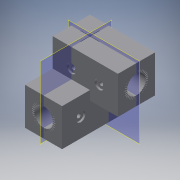
# Autodesk Inventor part: cam_holder_angle_part
Saved by Autodesk Inventor 2019 (Build 230136000, 136)
## iProperties
Created: 2024-08-06
Part Number: cam_holder_angle_part
Material: Generisch
Document SubType Name: Modeling
Designer: nic
Density: 1 g/cm^3
Appearance: Vorgabe
Author: nic
Autodesk Inventor part; units mm, degrees
ref_plane "YZ Plane" through (0, 0, 0) normal (1, 0, 0) x (0, 1, 0)
ref_plane "XZ Plane" through (0, 0, 0) normal (0, 1, 0) x (-1, 0, 0)
ref_plane "XY Plane" through (0, 0, 0) normal (0, 0, 1) x (1, 0, 0)
sketch "Skizze12" plane through (0, 0, 0) normal (0, 0, 1) x (1, 0, 0)
  circle A0 centre (0, 0) radius 10.1
  line L0 (-20, 20) -> (20, 20)
  line L1 (20, 20) -> (20, -20)
  line L2 (20, -20) -> (-20, -20)
  line L3 (-20, -20) -> (-20, 20)
  line L4 (-20, 20) -> (20, -20) construction
  line L5 (20, 20) -> (-20, -20) construction
  dimension "d59" = 20.2
  dimension "d60" = 40
  dimension "d61" = 40
  constraints: 12 end point, 2 midpoint, 2 parallel, 1 centre point, 1 coincident, 1 horizontal, 1 perpendicular
  measures "d59" diameter of A0
  measures "d60" distance of L1.end L2.end
  measures "d61" distance of L0.end L1.end
extrude "Extrusion10" add sketch "Skizze12" along normal blind 70
sketch "Skizze13" plane through (-20, -20, 0) normal (-1, 0, 0) x (0, 0, 1)
  line L0 (70, 30.1) -> (70, 9.9) projected
  line L1 (0, 9.9) -> (0, 30.1) projected
  line L2 (0, 30.1) -> (40, 30.1)
  line L3 (40, 30.1) -> (40, 70.1)
  line L4 (40, 70.1) -> (0, 70.1)
  line L5 (0, 70.1) -> (0, 30.1)
  circle A0 centre (20, 50.1) radius 10.1
  point P0 (0, 20)
  dimension "d64" = 40
  dimension "d65" = 40
  dimension "d66" = 20.2
  constraints: 8 end point, 2 parallel, 1 centre point, 1 horizontal, 1 perpendicular
  measures "d64" distance of L4.end L3.end
  measures "d65" distance of L3.end L2.end
  measures "d66" diameter of A0
extrude "Extrusion11" add sketch "Skizze13" against normal blind 70
sketch "Skizze14" plane through (-20, 20, 40) normal (0, 0, 1) x (1, 0, 0)
  line L0 (70, 20.2) -> (70, 0) projected
  line L1 (0, 0) -> (0, 20.2) projected
  line L2 (0, 0) -> (0, 20.2) projected
  line L3 (0, 10.1) -> (20, 10.1)
  line L4 (70, 20.2) -> (70, 0) projected
  line L5 (70, 10.1) -> (50, 10.1)
  point P0 (20, -20)
  dimension "d69" = 20
  dimension "d70" = 20
  constraints: 4 end point, 2 coincident, 2 midpoint, 1 horizontal, 1 point on line
  measures "d69" distance of L3.start L3.end
  measures "d70" distance of L5.start L5.end
hole "Bohrung3" at (0, 30.1, 40) at (30, 30.1, 40) direction (0, 0, -1) diameter 4.3 depth 12 tip angle 118 counterbore diameter 10 counterbore depth 2
sketch "Skizze15" plane through (20, -20, 70) normal (1, 0, 0) x (0, 0, -1)
  line L0 (0, 9.9) -> (0, 30.1) projected
  line L1 (70, 30.1) -> (70, 9.9) projected
  line L2 (0, 9.9) -> (0, 30.1) projected
  line L3 (0, 20) -> (20, 20)
  line L4 (70, 20) -> (50, 20)
  dimension "d78" = 20
  dimension "d79" = 20
  constraints: 4 end point, 2 coincident, 2 horizontal, 1 midpoint
  measures "d78" distance of L3.start L3.end
  measures "d79" distance of L4.start L4.end
hole "Bohrung4" at (20, 0, 50) at (20, 0, 20) direction (-1, 0, 0) diameter 4.3 depth 12 tip angle 118 counterbore diameter 10 counterbore depth 2
sketch "Skizze16" plane through (50, -20, 0) normal (1, 0, 0) x (0, 0, -1)
  circle A0 centre (-20, 50.1) radius 10.1 construction
  line L0 (-20.25, 57.7) -> (-19.75, 57.7)
  line L1 (-19.75, 57.7) -> (-19.75, 62.7)
  line L2 (-19.75, 62.7) -> (-20.25, 62.7)
  line L3 (-20.25, 62.7) -> (-20.25, 57.7)
  line L4 (-20.25, 57.7) -> (-19.75, 62.7) construction
  line L5 (-19.75, 57.7) -> (-20.25, 62.7) construction
  line L6 (-21.5659, 57.5411) -> (-21.0735, 57.628)
  line L7 (-21.0735, 57.628) -> (-21.9418, 62.552)
  line L8 (-21.9418, 62.552) -> (-22.4342, 62.4652)
  line L9 (-22.4342, 62.4652) -> (-21.5659, 57.5411)
  line L10 (-21.5659, 57.5411) -> (-21.9418, 62.552) construction
  line L11 (-21.0735, 57.628) -> (-22.4342, 62.4652) construction
  line L12 (-22.8343, 57.1562) -> (-22.3644, 57.3272)
  line L13 (-22.3644, 57.3272) -> (-24.0745, 62.0256)
  line L14 (-24.0745, 62.0256) -> (-24.5444, 61.8546)
  line L15 (-24.5444, 61.8546) -> (-22.8343, 57.1562)
  line L16 (-22.8343, 57.1562) -> (-24.0745, 62.0256) construction
  line L17 (-22.3644, 57.3272) -> (-24.5444, 61.8546) construction
  line L18 (-24.0165, 56.5568) -> (-23.5835, 56.8068)
  line L19 (-23.5835, 56.8068) -> (-26.0835, 61.1369)
  line L20 (-26.0835, 61.1369) -> (-26.5165, 60.8869)
  line L21 (-26.5165, 60.8869) -> (-24.0165, 56.5568)
  line L22 (-24.0165, 56.5568) -> (-26.0835, 61.1369) construction
  line L23 (-23.5835, 56.8068) -> (-26.5165, 60.8869) construction
  line L24 (-25.0767, 55.7612) -> (-24.6937, 56.0826)
  line L25 (-24.6937, 56.0826) -> (-27.9076, 59.9129)
  line L26 (-27.9076, 59.9129) -> (-28.2906, 59.5915)
  line L27 (-28.2906, 59.5915) -> (-25.0767, 55.7612)
  line L28 (-25.0767, 55.7612) -> (-27.9076, 59.9129) construction
  line L29 (-24.6937, 56.0826) -> (-28.2906, 59.5915) construction
  line L30 (-25.9826, 54.7937) -> (-25.6612, 55.1767)
  line L31 (-25.6612, 55.1767) -> (-29.4915, 58.3906)
  line L32 (-29.4915, 58.3906) -> (-29.8129, 58.0076)
  line L33 (-29.8129, 58.0076) -> (-25.9826, 54.7937)
  line L34 (-25.9826, 54.7937) -> (-29.4915, 58.3906) construction
  line L35 (-25.6612, 55.1767) -> (-29.8129, 58.0076) construction
  line L36 (-26.7068, 53.6835) -> (-26.4568, 54.1165)
  line L37 (-26.4568, 54.1165) -> (-30.7869, 56.6165)
  line L38 (-30.7869, 56.6165) -> (-31.0369, 56.1835)
  line L39 (-31.0369, 56.1835) -> (-26.7068, 53.6835)
  line L40 (-26.7068, 53.6835) -> (-30.7869, 56.6165) construction
  line L41 (-26.4568, 54.1165) -> (-31.0369, 56.1835) construction
  line L42 (-27.2272, 52.4644) -> (-27.0562, 52.9343)
  line L43 (-27.0562, 52.9343) -> (-31.7546, 54.6444)
  line L44 (-31.7546, 54.6444) -> (-31.9256, 54.1745)
  line L45 (-31.9256, 54.1745) -> (-27.2272, 52.4644)
  line L46 (-27.2272, 52.4644) -> (-31.7546, 54.6444) construction
  line L47 (-27.0562, 52.9343) -> (-31.9256, 54.1745) construction
  line L48 (-27.528, 51.1735) -> (-27.4411, 51.6659)
  line L49 (-27.4411, 51.6659) -> (-32.3652, 52.5342)
  line L50 (-32.3652, 52.5342) -> (-32.452, 52.0418)
  line L51 (-32.452, 52.0418) -> (-27.528, 51.1735)
  line L52 (-27.528, 51.1735) -> (-32.3652, 52.5342) construction
  line L53 (-27.4411, 51.6659) -> (-32.452, 52.0418) construction
  line L54 (-27.6, 49.85) -> (-27.6, 50.35)
  line L55 (-27.6, 50.35) -> (-32.6, 50.35)
  line L56 (-32.6, 50.35) -> (-32.6, 49.85)
  line L57 (-32.6, 49.85) -> (-27.6, 49.85)
  line L58 (-27.6, 49.85) -> (-32.6, 50.35) construction
  line L59 (-27.6, 50.35) -> (-32.6, 49.85) construction
  line L60 (-27.4411, 48.5341) -> (-27.528, 49.0265)
  line L61 (-27.528, 49.0265) -> (-32.452, 48.1582)
  line L62 (-32.452, 48.1582) -> (-32.3652, 47.6658)
  line L63 (-32.3652, 47.6658) -> (-27.4411, 48.5341)
  line L64 (-27.4411, 48.5341) -> (-32.452, 48.1582) construction
  line L65 (-27.528, 49.0265) -> (-32.3652, 47.6658) construction
  line L66 (-27.0562, 47.2657) -> (-27.2272, 47.7356)
  line L67 (-27.2272, 47.7356) -> (-31.9256, 46.0255)
  line L68 (-31.9256, 46.0255) -> (-31.7546, 45.5556)
  line L69 (-31.7546, 45.5556) -> (-27.0562, 47.2657)
  line L70 (-27.0562, 47.2657) -> (-31.9256, 46.0255) construction
  line L71 (-27.2272, 47.7356) -> (-31.7546, 45.5556) construction
  line L72 (-26.4568, 46.0835) -> (-26.7068, 46.5165)
  line L73 (-26.7068, 46.5165) -> (-31.0369, 44.0165)
  line L74 (-31.0369, 44.0165) -> (-30.7869, 43.5835)
  line L75 (-30.7869, 43.5835) -> (-26.4568, 46.0835)
  line L76 (-26.4568, 46.0835) -> (-31.0369, 44.0165) construction
  line L77 (-26.7068, 46.5165) -> (-30.7869, 43.5835) construction
  line L78 (-25.6612, 45.0233) -> (-25.9826, 45.4063)
  line L79 (-25.9826, 45.4063) -> (-29.8129, 42.1924)
  line L80 (-29.8129, 42.1924) -> (-29.4915, 41.8094)
  line L81 (-29.4915, 41.8094) -> (-25.6612, 45.0233)
  line L82 (-25.6612, 45.0233) -> (-29.8129, 42.1924) construction
  line L83 (-25.9826, 45.4063) -> (-29.4915, 41.8094) construction
  line L84 (-24.6937, 44.1174) -> (-25.0767, 44.4388)
  line L85 (-25.0767, 44.4388) -> (-28.2906, 40.6085)
  line L86 (-28.2906, 40.6085) -> (-27.9076, 40.2871)
  line L87 (-27.9076, 40.2871) -> (-24.6937, 44.1174)
  line L88 (-24.6937, 44.1174) -> (-28.2906, 40.6085) construction
  line L89 (-25.0767, 44.4388) -> (-27.9076, 40.2871) construction
  line L90 (-23.5835, 43.3932) -> (-24.0165, 43.6432)
  line L91 (-24.0165, 43.6432) -> (-26.5165, 39.3131)
  line L92 (-26.5165, 39.3131) -> (-26.0835, 39.0631)
  line L93 (-26.0835, 39.0631) -> (-23.5835, 43.3932)
  line L94 (-23.5835, 43.3932) -> (-26.5165, 39.3131) construction
  line L95 (-24.0165, 43.6432) -> (-26.0835, 39.0631) construction
  line L96 (-22.3644, 42.8728) -> (-22.8343, 43.0438)
  line L97 (-22.8343, 43.0438) -> (-24.5444, 38.3454)
  line L98 (-24.5444, 38.3454) -> (-24.0745, 38.1744)
  line L99 (-24.0745, 38.1744) -> (-22.3644, 42.8728)
  line L100 (-22.3644, 42.8728) -> (-24.5444, 38.3454) construction
  line L101 (-22.8343, 43.0438) -> (-24.0745, 38.1744) construction
  line L102 (-21.0735, 42.572) -> (-21.5659, 42.6589)
  line L103 (-21.5659, 42.6589) -> (-22.4342, 37.7348)
  line L104 (-22.4342, 37.7348) -> (-21.9418, 37.648)
  line L105 (-21.9418, 37.648) -> (-21.0735, 42.572)
  line L106 (-21.0735, 42.572) -> (-22.4342, 37.7348) construction
  line L107 (-21.5659, 42.6589) -> (-21.9418, 37.648) construction
  line L108 (-19.75, 42.5) -> (-20.25, 42.5)
  line L109 (-20.25, 42.5) -> (-20.25, 37.5)
  line L110 (-20.25, 37.5) -> (-19.75, 37.5)
  line L111 (-19.75, 37.5) -> (-19.75, 42.5)
  line L112 (-19.75, 42.5) -> (-20.25, 37.5) construction
  line L113 (-20.25, 42.5) -> (-19.75, 37.5) construction
  line L114 (-18.4341, 42.6589) -> (-18.9265, 42.572)
  line L115 (-18.9265, 42.572) -> (-18.0582, 37.648)
  line L116 (-18.0582, 37.648) -> (-17.5658, 37.7348)
  line L117 (-17.5658, 37.7348) -> (-18.4341, 42.6589)
  line L118 (-18.4341, 42.6589) -> (-18.0582, 37.648) construction
  line L119 (-18.9265, 42.572) -> (-17.5658, 37.7348) construction
  line L120 (-17.1657, 43.0438) -> (-17.6356, 42.8728)
  line L121 (-17.6356, 42.8728) -> (-15.9255, 38.1744)
  line L122 (-15.9255, 38.1744) -> (-15.4556, 38.3454)
  line L123 (-15.4556, 38.3454) -> (-17.1657, 43.0438)
  line L124 (-17.1657, 43.0438) -> (-15.9255, 38.1744) construction
  line L125 (-17.6356, 42.8728) -> (-15.4556, 38.3454) construction
  line L126 (-15.9835, 43.6432) -> (-16.4165, 43.3932)
  line L127 (-16.4165, 43.3932) -> (-13.9165, 39.0631)
  line L128 (-13.9165, 39.0631) -> (-13.4835, 39.3131)
  line L129 (-13.4835, 39.3131) -> (-15.9835, 43.6432)
  line L130 (-15.9835, 43.6432) -> (-13.9165, 39.0631) construction
  line L131 (-16.4165, 43.3932) -> (-13.4835, 39.3131) construction
  line L132 (-14.9233, 44.4388) -> (-15.3063, 44.1174)
  line L133 (-15.3063, 44.1174) -> (-12.0924, 40.2871)
  line L134 (-12.0924, 40.2871) -> (-11.7094, 40.6085)
  line L135 (-11.7094, 40.6085) -> (-14.9233, 44.4388)
  line L136 (-14.9233, 44.4388) -> (-12.0924, 40.2871) construction
  line L137 (-15.3063, 44.1174) -> (-11.7094, 40.6085) construction
  line L138 (-14.0174, 45.4063) -> (-14.3388, 45.0233)
  line L139 (-14.3388, 45.0233) -> (-10.5085, 41.8094)
  line L140 (-10.5085, 41.8094) -> (-10.1871, 42.1924)
  line L141 (-10.1871, 42.1924) -> (-14.0174, 45.4063)
  line L142 (-14.0174, 45.4063) -> (-10.5085, 41.8094) construction
  line L143 (-14.3388, 45.0233) -> (-10.1871, 42.1924) construction
  line L144 (-13.2932, 46.5165) -> (-13.5432, 46.0835)
  line L145 (-13.5432, 46.0835) -> (-9.2131, 43.5835)
  line L146 (-9.2131, 43.5835) -> (-8.9631, 44.0165)
  line L147 (-8.9631, 44.0165) -> (-13.2932, 46.5165)
  line L148 (-13.2932, 46.5165) -> (-9.2131, 43.5835) construction
  line L149 (-13.5432, 46.0835) -> (-8.9631, 44.0165) construction
  line L150 (-12.7728, 47.7356) -> (-12.9438, 47.2657)
  line L151 (-12.9438, 47.2657) -> (-8.2454, 45.5556)
  line L152 (-8.2454, 45.5556) -> (-8.0744, 46.0255)
  line L153 (-8.0744, 46.0255) -> (-12.7728, 47.7356)
  line L154 (-12.7728, 47.7356) -> (-8.2454, 45.5556) construction
  line L155 (-12.9438, 47.2657) -> (-8.0744, 46.0255) construction
  line L156 (-12.472, 49.0265) -> (-12.5589, 48.5341)
  line L157 (-12.5589, 48.5341) -> (-7.6348, 47.6658)
  line L158 (-7.6348, 47.6658) -> (-7.548, 48.1582)
  line L159 (-7.548, 48.1582) -> (-12.472, 49.0265)
  line L160 (-12.472, 49.0265) -> (-7.6348, 47.6658) construction
  line L161 (-12.5589, 48.5341) -> (-7.548, 48.1582) construction
  line L162 (-12.4, 50.35) -> (-12.4, 49.85)
  line L163 (-12.4, 49.85) -> (-7.4, 49.85)
  line L164 (-7.4, 49.85) -> (-7.4, 50.35)
  line L165 (-7.4, 50.35) -> (-12.4, 50.35)
  line L166 (-12.4, 50.35) -> (-7.4, 49.85) construction
  line L167 (-12.4, 49.85) -> (-7.4, 50.35) construction
  line L168 (-12.5589, 51.6659) -> (-12.472, 51.1735)
  line L169 (-12.472, 51.1735) -> (-7.548, 52.0418)
  line L170 (-7.548, 52.0418) -> (-7.6348, 52.5342)
  line L171 (-7.6348, 52.5342) -> (-12.5589, 51.6659)
  line L172 (-12.5589, 51.6659) -> (-7.548, 52.0418) construction
  line L173 (-12.472, 51.1735) -> (-7.6348, 52.5342) construction
  line L174 (-12.9438, 52.9343) -> (-12.7728, 52.4644)
  line L175 (-12.7728, 52.4644) -> (-8.0744, 54.1745)
  line L176 (-8.0744, 54.1745) -> (-8.2454, 54.6444)
  line L177 (-8.2454, 54.6444) -> (-12.9438, 52.9343)
  line L178 (-12.9438, 52.9343) -> (-8.0744, 54.1745) construction
  line L179 (-12.7728, 52.4644) -> (-8.2454, 54.6444) construction
  line L180 (-13.5432, 54.1165) -> (-13.2932, 53.6835)
  line L181 (-13.2932, 53.6835) -> (-8.9631, 56.1835)
  line L182 (-8.9631, 56.1835) -> (-9.2131, 56.6165)
  line L183 (-9.2131, 56.6165) -> (-13.5432, 54.1165)
  line L184 (-13.5432, 54.1165) -> (-8.9631, 56.1835) construction
  line L185 (-13.2932, 53.6835) -> (-9.2131, 56.6165) construction
  line L186 (-14.3388, 55.1767) -> (-14.0174, 54.7937)
  line L187 (-14.0174, 54.7937) -> (-10.1871, 58.0076)
  line L188 (-10.1871, 58.0076) -> (-10.5085, 58.3906)
  line L189 (-10.5085, 58.3906) -> (-14.3388, 55.1767)
  line L190 (-14.3388, 55.1767) -> (-10.1871, 58.0076) construction
  line L191 (-14.0174, 54.7937) -> (-10.5085, 58.3906) construction
  line L192 (-15.3063, 56.0826) -> (-14.9233, 55.7612)
  line L193 (-14.9233, 55.7612) -> (-11.7094, 59.5915)
  line L194 (-11.7094, 59.5915) -> (-12.0924, 59.9129)
  line L195 (-12.0924, 59.9129) -> (-15.3063, 56.0826)
  line L196 (-15.3063, 56.0826) -> (-11.7094, 59.5915) construction
  line L197 (-14.9233, 55.7612) -> (-12.0924, 59.9129) construction
  line L198 (-16.4165, 56.8068) -> (-15.9835, 56.5568)
  line L199 (-15.9835, 56.5568) -> (-13.4835, 60.8869)
  line L200 (-13.4835, 60.8869) -> (-13.9165, 61.1369)
  line L201 (-13.9165, 61.1369) -> (-16.4165, 56.8068)
  line L202 (-16.4165, 56.8068) -> (-13.4835, 60.8869) construction
  line L203 (-15.9835, 56.5568) -> (-13.9165, 61.1369) construction
  line L204 (-17.6356, 57.3272) -> (-17.1657, 57.1562)
  line L205 (-17.1657, 57.1562) -> (-15.4556, 61.8546)
  line L206 (-15.4556, 61.8546) -> (-15.9255, 62.0256)
  line L207 (-15.9255, 62.0256) -> (-17.6356, 57.3272)
  line L208 (-17.6356, 57.3272) -> (-15.4556, 61.8546) construction
  line L209 (-17.1657, 57.1562) -> (-15.9255, 62.0256) construction
  line L210 (-18.9265, 57.628) -> (-18.4341, 57.5411)
  line L211 (-18.4341, 57.5411) -> (-17.5658, 62.4652)
  line L212 (-17.5658, 62.4652) -> (-18.0582, 62.552)
  line L213 (-18.0582, 62.552) -> (-18.9265, 57.628)
  line L214 (-18.9265, 57.628) -> (-17.5658, 62.4652) construction
  line L215 (-18.4341, 57.5411) -> (-18.0582, 62.552) construction
  line L216 (-20.25, 35.1) -> (-19.75, 35.1)
  line L217 (-19.75, 35.1) -> (-19.75, 65.1)
  line L218 (-19.75, 65.1) -> (-20.25, 65.1)
  line L219 (-20.25, 65.1) -> (-20.25, 35.1)
  line L220 (-20.25, 35.1) -> (-19.75, 65.1) construction
  line L221 (-19.75, 35.1) -> (-20.25, 65.1) construction
  point P0 (0, 20)
  point P1 (-20, 60.2)
  point P2 (-21.7538, 60.0466)
  point P3 (-23.4544, 59.5909)
  point P4 (-25.05, 58.8469)
  point P5 (-26.4922, 57.837)
  point P6 (-27.737, 56.5922)
  point P7 (-28.7469, 55.15)
  point P8 (-29.4909, 53.5544)
  point P9 (-29.9466, 51.8538)
  point P10 (-30.1, 50.1)
  point P11 (-29.9466, 48.3462)
  point P12 (-29.4909, 46.6456)
  point P13 (-28.7469, 45.05)
  point P14 (-27.737, 43.6078)
  point P15 (-26.4922, 42.363)
  point P16 (-25.05, 41.3531)
  point P17 (-23.4544, 40.6091)
  point P18 (-21.7538, 40.1534)
  point P19 (-20, 40)
  point P20 (-18.2462, 40.1534)
  point P21 (-16.5456, 40.6091)
  point P22 (-14.95, 41.3531)
  point P23 (-13.5078, 42.363)
  point P24 (-12.263, 43.6078)
  point P25 (-11.2531, 45.05)
  point P26 (-10.5091, 46.6456)
  point P27 (-10.0534, 48.3462)
  point P28 (-9.9, 50.1)
  point P29 (-10.0534, 51.8538)
  point P30 (-10.5091, 53.5544)
  point P31 (-11.2531, 55.15)
  point P32 (-12.263, 56.5922)
  point P33 (-13.5078, 57.837)
  point P34 (-14.95, 58.8469)
  point P35 (-16.5456, 59.5909)
  point P36 (-18.2462, 60.0466)
  dimension "d87" = 0.5
  dimension "d88" = 5
  dimension "d91" = 360
  dimension "d93" = 30
  constraints: 444 end point, 74 midpoint, 4 parallel, 2 horizontal, 2 perpendicular, 1 point on line, 1 vertical alignment, 398 other
  measures "d87" distance of L2.end L1.end
  measures "d88" distance of L1.end L0.end
  measures "d93" distance of L217.end L216.end
extrude "Extrusion12" cut sketch "Skizze16" against normal blind 0.5
sketch "Skizze18" plane through (0, 0, 70) normal (0, 0, 1) x (1, 0, 0)
  circle A0 centre (0, 0) radius 10.1 construction
  line L0 (-0.25, 7.6) -> (0.25, 7.6)
  line L1 (0.25, 7.6) -> (0.25, 12.6)
  line L2 (0.25, 12.6) -> (-0.25, 12.6)
  line L3 (-0.25, 12.6) -> (-0.25, 7.6)
  line L4 (-0.25, 7.6) -> (0.25, 12.6) construction
  line L5 (0.25, 7.6) -> (-0.25, 12.6) construction
  line L6 (-1.5659, 7.4411) -> (-1.0735, 7.528)
  line L7 (-1.0735, 7.528) -> (-1.9418, 12.452)
  line L8 (-1.9418, 12.452) -> (-2.4342, 12.3652)
  line L9 (-2.4342, 12.3652) -> (-1.5659, 7.4411)
  line L10 (-1.5659, 7.4411) -> (-1.9418, 12.452) construction
  line L11 (-1.0735, 7.528) -> (-2.4342, 12.3652) construction
  line L12 (-2.8343, 7.0562) -> (-2.3644, 7.2272)
  line L13 (-2.3644, 7.2272) -> (-4.0745, 11.9256)
  line L14 (-4.0745, 11.9256) -> (-4.5444, 11.7546)
  line L15 (-4.5444, 11.7546) -> (-2.8343, 7.0562)
  line L16 (-2.8343, 7.0562) -> (-4.0745, 11.9256) construction
  line L17 (-2.3644, 7.2272) -> (-4.5444, 11.7546) construction
  line L18 (-4.0165, 6.4568) -> (-3.5835, 6.7068)
  line L19 (-3.5835, 6.7068) -> (-6.0835, 11.0369)
  line L20 (-6.0835, 11.0369) -> (-6.5165, 10.7869)
  line L21 (-6.5165, 10.7869) -> (-4.0165, 6.4568)
  line L22 (-4.0165, 6.4568) -> (-6.0835, 11.0369) construction
  line L23 (-3.5835, 6.7068) -> (-6.5165, 10.7869) construction
  line L24 (-5.0767, 5.6612) -> (-4.6937, 5.9826)
  line L25 (-4.6937, 5.9826) -> (-7.9076, 9.8129)
  line L26 (-7.9076, 9.8129) -> (-8.2906, 9.4915)
  line L27 (-8.2906, 9.4915) -> (-5.0767, 5.6612)
  line L28 (-5.0767, 5.6612) -> (-7.9076, 9.8129) construction
  line L29 (-4.6937, 5.9826) -> (-8.2906, 9.4915) construction
  line L30 (-5.9826, 4.6937) -> (-5.6612, 5.0767)
  line L31 (-5.6612, 5.0767) -> (-9.4915, 8.2906)
  line L32 (-9.4915, 8.2906) -> (-9.8129, 7.9076)
  line L33 (-9.8129, 7.9076) -> (-5.9826, 4.6937)
  line L34 (-5.9826, 4.6937) -> (-9.4915, 8.2906) construction
  line L35 (-5.6612, 5.0767) -> (-9.8129, 7.9076) construction
  line L36 (-6.7068, 3.5835) -> (-6.4568, 4.0165)
  line L37 (-6.4568, 4.0165) -> (-10.7869, 6.5165)
  line L38 (-10.7869, 6.5165) -> (-11.0369, 6.0835)
  line L39 (-11.0369, 6.0835) -> (-6.7068, 3.5835)
  line L40 (-6.7068, 3.5835) -> (-10.7869, 6.5165) construction
  line L41 (-6.4568, 4.0165) -> (-11.0369, 6.0835) construction
  line L42 (-7.2272, 2.3644) -> (-7.0562, 2.8343)
  line L43 (-7.0562, 2.8343) -> (-11.7546, 4.5444)
  line L44 (-11.7546, 4.5444) -> (-11.9256, 4.0745)
  line L45 (-11.9256, 4.0745) -> (-7.2272, 2.3644)
  line L46 (-7.2272, 2.3644) -> (-11.7546, 4.5444) construction
  line L47 (-7.0562, 2.8343) -> (-11.9256, 4.0745) construction
  line L48 (-7.528, 1.0735) -> (-7.4411, 1.5659)
  line L49 (-7.4411, 1.5659) -> (-12.3652, 2.4342)
  line L50 (-12.3652, 2.4342) -> (-12.452, 1.9418)
  line L51 (-12.452, 1.9418) -> (-7.528, 1.0735)
  line L52 (-7.528, 1.0735) -> (-12.3652, 2.4342) construction
  line L53 (-7.4411, 1.5659) -> (-12.452, 1.9418) construction
  line L54 (-7.6, -0.25) -> (-7.6, 0.25)
  line L55 (-7.6, 0.25) -> (-12.6, 0.25)
  line L56 (-12.6, 0.25) -> (-12.6, -0.25)
  line L57 (-12.6, -0.25) -> (-7.6, -0.25)
  line L58 (-7.6, -0.25) -> (-12.6, 0.25) construction
  line L59 (-7.6, 0.25) -> (-12.6, -0.25) construction
  line L60 (-7.4411, -1.5659) -> (-7.528, -1.0735)
  line L61 (-7.528, -1.0735) -> (-12.452, -1.9418)
  line L62 (-12.452, -1.9418) -> (-12.3652, -2.4342)
  line L63 (-12.3652, -2.4342) -> (-7.4411, -1.5659)
  line L64 (-7.4411, -1.5659) -> (-12.452, -1.9418) construction
  line L65 (-7.528, -1.0735) -> (-12.3652, -2.4342) construction
  line L66 (-7.0562, -2.8343) -> (-7.2272, -2.3644)
  line L67 (-7.2272, -2.3644) -> (-11.9256, -4.0745)
  line L68 (-11.9256, -4.0745) -> (-11.7546, -4.5444)
  line L69 (-11.7546, -4.5444) -> (-7.0562, -2.8343)
  line L70 (-7.0562, -2.8343) -> (-11.9256, -4.0745) construction
  line L71 (-7.2272, -2.3644) -> (-11.7546, -4.5444) construction
  line L72 (-6.4568, -4.0165) -> (-6.7068, -3.5835)
  line L73 (-6.7068, -3.5835) -> (-11.0369, -6.0835)
  line L74 (-11.0369, -6.0835) -> (-10.7869, -6.5165)
  line L75 (-10.7869, -6.5165) -> (-6.4568, -4.0165)
  line L76 (-6.4568, -4.0165) -> (-11.0369, -6.0835) construction
  line L77 (-6.7068, -3.5835) -> (-10.7869, -6.5165) construction
  line L78 (-5.6612, -5.0767) -> (-5.9826, -4.6937)
  line L79 (-5.9826, -4.6937) -> (-9.8129, -7.9076)
  line L80 (-9.8129, -7.9076) -> (-9.4915, -8.2906)
  line L81 (-9.4915, -8.2906) -> (-5.6612, -5.0767)
  line L82 (-5.6612, -5.0767) -> (-9.8129, -7.9076) construction
  line L83 (-5.9826, -4.6937) -> (-9.4915, -8.2906) construction
  line L84 (-4.6937, -5.9826) -> (-5.0767, -5.6612)
  line L85 (-5.0767, -5.6612) -> (-8.2906, -9.4915)
  line L86 (-8.2906, -9.4915) -> (-7.9076, -9.8129)
  line L87 (-7.9076, -9.8129) -> (-4.6937, -5.9826)
  line L88 (-4.6937, -5.9826) -> (-8.2906, -9.4915) construction
  line L89 (-5.0767, -5.6612) -> (-7.9076, -9.8129) construction
  line L90 (-3.5835, -6.7068) -> (-4.0165, -6.4568)
  line L91 (-4.0165, -6.4568) -> (-6.5165, -10.7869)
  line L92 (-6.5165, -10.7869) -> (-6.0835, -11.0369)
  line L93 (-6.0835, -11.0369) -> (-3.5835, -6.7068)
  line L94 (-3.5835, -6.7068) -> (-6.5165, -10.7869) construction
  line L95 (-4.0165, -6.4568) -> (-6.0835, -11.0369) construction
  line L96 (-2.3644, -7.2272) -> (-2.8343, -7.0562)
  line L97 (-2.8343, -7.0562) -> (-4.5444, -11.7546)
  line L98 (-4.5444, -11.7546) -> (-4.0745, -11.9256)
  line L99 (-4.0745, -11.9256) -> (-2.3644, -7.2272)
  line L100 (-2.3644, -7.2272) -> (-4.5444, -11.7546) construction
  line L101 (-2.8343, -7.0562) -> (-4.0745, -11.9256) construction
  line L102 (-1.0735, -7.528) -> (-1.5659, -7.4411)
  line L103 (-1.5659, -7.4411) -> (-2.4342, -12.3652)
  line L104 (-2.4342, -12.3652) -> (-1.9418, -12.452)
  line L105 (-1.9418, -12.452) -> (-1.0735, -7.528)
  line L106 (-1.0735, -7.528) -> (-2.4342, -12.3652) construction
  line L107 (-1.5659, -7.4411) -> (-1.9418, -12.452) construction
  line L108 (0.25, -7.6) -> (-0.25, -7.6)
  line L109 (-0.25, -7.6) -> (-0.25, -12.6)
  line L110 (-0.25, -12.6) -> (0.25, -12.6)
  line L111 (0.25, -12.6) -> (0.25, -7.6)
  line L112 (0.25, -7.6) -> (-0.25, -12.6) construction
  line L113 (-0.25, -7.6) -> (0.25, -12.6) construction
  line L114 (1.5659, -7.4411) -> (1.0735, -7.528)
  line L115 (1.0735, -7.528) -> (1.9418, -12.452)
  line L116 (1.9418, -12.452) -> (2.4342, -12.3652)
  line L117 (2.4342, -12.3652) -> (1.5659, -7.4411)
  line L118 (1.5659, -7.4411) -> (1.9418, -12.452) construction
  line L119 (1.0735, -7.528) -> (2.4342, -12.3652) construction
  line L120 (2.8343, -7.0562) -> (2.3644, -7.2272)
  line L121 (2.3644, -7.2272) -> (4.0745, -11.9256)
  line L122 (4.0745, -11.9256) -> (4.5444, -11.7546)
  line L123 (4.5444, -11.7546) -> (2.8343, -7.0562)
  line L124 (2.8343, -7.0562) -> (4.0745, -11.9256) construction
  line L125 (2.3644, -7.2272) -> (4.5444, -11.7546) construction
  line L126 (4.0165, -6.4568) -> (3.5835, -6.7068)
  line L127 (3.5835, -6.7068) -> (6.0835, -11.0369)
  line L128 (6.0835, -11.0369) -> (6.5165, -10.7869)
  line L129 (6.5165, -10.7869) -> (4.0165, -6.4568)
  line L130 (4.0165, -6.4568) -> (6.0835, -11.0369) construction
  line L131 (3.5835, -6.7068) -> (6.5165, -10.7869) construction
  line L132 (5.0767, -5.6612) -> (4.6937, -5.9826)
  line L133 (4.6937, -5.9826) -> (7.9076, -9.8129)
  line L134 (7.9076, -9.8129) -> (8.2906, -9.4915)
  line L135 (8.2906, -9.4915) -> (5.0767, -5.6612)
  line L136 (5.0767, -5.6612) -> (7.9076, -9.8129) construction
  line L137 (4.6937, -5.9826) -> (8.2906, -9.4915) construction
  line L138 (5.9826, -4.6937) -> (5.6612, -5.0767)
  line L139 (5.6612, -5.0767) -> (9.4915, -8.2906)
  line L140 (9.4915, -8.2906) -> (9.8129, -7.9076)
  line L141 (9.8129, -7.9076) -> (5.9826, -4.6937)
  line L142 (5.9826, -4.6937) -> (9.4915, -8.2906) construction
  line L143 (5.6612, -5.0767) -> (9.8129, -7.9076) construction
  line L144 (6.7068, -3.5835) -> (6.4568, -4.0165)
  line L145 (6.4568, -4.0165) -> (10.7869, -6.5165)
  line L146 (10.7869, -6.5165) -> (11.0369, -6.0835)
  line L147 (11.0369, -6.0835) -> (6.7068, -3.5835)
  line L148 (6.7068, -3.5835) -> (10.7869, -6.5165) construction
  line L149 (6.4568, -4.0165) -> (11.0369, -6.0835) construction
  line L150 (7.2272, -2.3644) -> (7.0562, -2.8343)
  line L151 (7.0562, -2.8343) -> (11.7546, -4.5444)
  line L152 (11.7546, -4.5444) -> (11.9256, -4.0745)
  line L153 (11.9256, -4.0745) -> (7.2272, -2.3644)
  line L154 (7.2272, -2.3644) -> (11.7546, -4.5444) construction
  line L155 (7.0562, -2.8343) -> (11.9256, -4.0745) construction
  line L156 (7.528, -1.0735) -> (7.4411, -1.5659)
  line L157 (7.4411, -1.5659) -> (12.3652, -2.4342)
  line L158 (12.3652, -2.4342) -> (12.452, -1.9418)
  line L159 (12.452, -1.9418) -> (7.528, -1.0735)
  line L160 (7.528, -1.0735) -> (12.3652, -2.4342) construction
  line L161 (7.4411, -1.5659) -> (12.452, -1.9418) construction
  line L162 (7.6, 0.25) -> (7.6, -0.25)
  line L163 (7.6, -0.25) -> (12.6, -0.25)
  line L164 (12.6, -0.25) -> (12.6, 0.25)
  line L165 (12.6, 0.25) -> (7.6, 0.25)
  line L166 (7.6, 0.25) -> (12.6, -0.25) construction
  line L167 (7.6, -0.25) -> (12.6, 0.25) construction
  line L168 (7.4411, 1.5659) -> (7.528, 1.0735)
  line L169 (7.528, 1.0735) -> (12.452, 1.9418)
  line L170 (12.452, 1.9418) -> (12.3652, 2.4342)
  line L171 (12.3652, 2.4342) -> (7.4411, 1.5659)
  line L172 (7.4411, 1.5659) -> (12.452, 1.9418) construction
  line L173 (7.528, 1.0735) -> (12.3652, 2.4342) construction
  line L174 (7.0562, 2.8343) -> (7.2272, 2.3644)
  line L175 (7.2272, 2.3644) -> (11.9256, 4.0745)
  line L176 (11.9256, 4.0745) -> (11.7546, 4.5444)
  line L177 (11.7546, 4.5444) -> (7.0562, 2.8343)
  line L178 (7.0562, 2.8343) -> (11.9256, 4.0745) construction
  line L179 (7.2272, 2.3644) -> (11.7546, 4.5444) construction
  line L180 (6.4568, 4.0165) -> (6.7068, 3.5835)
  line L181 (6.7068, 3.5835) -> (11.0369, 6.0835)
  line L182 (11.0369, 6.0835) -> (10.7869, 6.5165)
  line L183 (10.7869, 6.5165) -> (6.4568, 4.0165)
  line L184 (6.4568, 4.0165) -> (11.0369, 6.0835) construction
  line L185 (6.7068, 3.5835) -> (10.7869, 6.5165) construction
  line L186 (5.6612, 5.0767) -> (5.9826, 4.6937)
  line L187 (5.9826, 4.6937) -> (9.8129, 7.9076)
  line L188 (9.8129, 7.9076) -> (9.4915, 8.2906)
  line L189 (9.4915, 8.2906) -> (5.6612, 5.0767)
  line L190 (5.6612, 5.0767) -> (9.8129, 7.9076) construction
  line L191 (5.9826, 4.6937) -> (9.4915, 8.2906) construction
  line L192 (4.6937, 5.9826) -> (5.0767, 5.6612)
  line L193 (5.0767, 5.6612) -> (8.2906, 9.4915)
  line L194 (8.2906, 9.4915) -> (7.9076, 9.8129)
  line L195 (7.9076, 9.8129) -> (4.6937, 5.9826)
  line L196 (4.6937, 5.9826) -> (8.2906, 9.4915) construction
  line L197 (5.0767, 5.6612) -> (7.9076, 9.8129) construction
  line L198 (3.5835, 6.7068) -> (4.0165, 6.4568)
  line L199 (4.0165, 6.4568) -> (6.5165, 10.7869)
  line L200 (6.5165, 10.7869) -> (6.0835, 11.0369)
  line L201 (6.0835, 11.0369) -> (3.5835, 6.7068)
  line L202 (3.5835, 6.7068) -> (6.5165, 10.7869) construction
  line L203 (4.0165, 6.4568) -> (6.0835, 11.0369) construction
  line L204 (2.3644, 7.2272) -> (2.8343, 7.0562)
  line L205 (2.8343, 7.0562) -> (4.5444, 11.7546)
  line L206 (4.5444, 11.7546) -> (4.0745, 11.9256)
  line L207 (4.0745, 11.9256) -> (2.3644, 7.2272)
  line L208 (2.3644, 7.2272) -> (4.5444, 11.7546) construction
  line L209 (2.8343, 7.0562) -> (4.0745, 11.9256) construction
  line L210 (1.0735, 7.528) -> (1.5659, 7.4411)
  line L211 (1.5659, 7.4411) -> (2.4342, 12.3652)
  line L212 (2.4342, 12.3652) -> (1.9418, 12.452)
  line L213 (1.9418, 12.452) -> (1.0735, 7.528)
  line L214 (1.0735, 7.528) -> (2.4342, 12.3652) construction
  line L215 (1.5659, 7.4411) -> (1.9418, 12.452) construction
  line L216 (-0.25, 15) -> (0.25, 15)
  line L217 (0.25, 15) -> (0.25, -15)
  line L218 (0.25, -15) -> (-0.25, -15)
  line L219 (-0.25, -15) -> (-0.25, 15)
  line L220 (-0.25, 15) -> (0.25, -15) construction
  line L221 (0.25, 15) -> (-0.25, -15) construction
  point P0 (0, 10.1)
  point P1 (-1.7538, 9.9466)
  point P2 (-3.4544, 9.4909)
  point P3 (-5.05, 8.7469)
  point P4 (-6.4922, 7.737)
  point P5 (-7.737, 6.4922)
  point P6 (-8.7469, 5.05)
  point P7 (-9.4909, 3.4544)
  point P8 (-9.9466, 1.7538)
  point P9 (-10.1, 0)
  point P10 (-9.9466, -1.7538)
  point P11 (-9.4909, -3.4544)
  point P12 (-8.7469, -5.05)
  point P13 (-7.737, -6.4922)
  point P14 (-6.4922, -7.737)
  point P15 (-5.05, -8.7469)
  point P16 (-3.4544, -9.4909)
  point P17 (-1.7538, -9.9466)
  point P18 (0, -10.1)
  point P19 (1.7538, -9.9466)
  point P20 (3.4544, -9.4909)
  point P21 (5.05, -8.7469)
  point P22 (6.4922, -7.737)
  point P23 (7.737, -6.4922)
  point P24 (8.7469, -5.05)
  point P25 (9.4909, -3.4544)
  point P26 (9.9466, -1.7538)
  point P27 (10.1, 0)
  point P28 (9.9466, 1.7538)
  point P29 (9.4909, 3.4544)
  point P30 (8.7469, 5.05)
  point P31 (7.737, 6.4922)
  point P32 (6.4922, 7.737)
  point P33 (5.05, 8.7469)
  point P34 (3.4544, 9.4909)
  point P35 (1.7538, 9.9466)
  dimension "d106" = 0.5
  dimension "d107" = 5
  dimension "d110" = 360
  dimension "d112" = 0.5
  dimension "d113" = 30
  constraints: 444 end point, 74 midpoint, 4 parallel, 2 horizontal, 2 perpendicular, 1 vertical alignment, 398 other
  measures "d106" distance of L2.end L1.end
  measures "d107" distance of L1.end L0.end
  measures "d112" distance of L217.end L218.end
  measures "d113" distance of L216.end L217.end
extrude "Extrusion14" cut sketch "Skizze18" against normal blind 0.5
sketch "Skizze20" plane through (-20, 50.1, 40) normal (0, 1, 0) x (1, 0, 0)
  line L0 (9.9, 40) -> (9.9, -29.5) projected
  line L1 (30.1, 40) -> (30.1, -29.5) projected
  line L2 (0, 30.1) -> (69.5, 30.1) projected
  line L3 (0, 9.9) -> (69.5, 9.9) projected
  line L4 (0, 30.1) -> (0, 20)
  line L5 (0, 40) -> (0, -30) projected
  line L6 (30, 19.75) -> (10, 19.75)
  line L7 (10, 19.75) -> (10, 20.25)
  line L8 (10, 20.25) -> (30, 20.25)
  line L9 (30, 20.25) -> (30, 19.75)
  line L10 (30, 19.75) -> (10, 20.25) construction
  line L11 (10, 19.75) -> (30, 20.25) construction
  line L12 (20.25, 30.1) -> (19.75, 30.1)
  line L13 (19.75, 30.1) -> (19.75, 9.9)
  line L14 (19.75, 9.9) -> (20.25, 9.9)
  line L15 (20.25, 9.9) -> (20.25, 30.1)
  line L16 (20.25, 30.1) -> (19.75, 9.9) construction
  line L17 (19.75, 30.1) -> (20.25, 9.9) construction
  point P0 (20, 40)
  point P1 (20, 20)
  dimension "d116" = 10.1
  dimension "d117" = 20
  dimension "d118" = 0.5
  dimension "d119" = 0.5
  constraints: 26 end point, 4 midpoint, 4 parallel, 2 horizontal, 2 perpendicular, 2 point on line
  measures "d116" distance of L2.start L4.end
  measures "d117" distance of L7.end L8.end
  measures "d118" distance of L6.end L7.end
  measures "d119" distance of L14.end L13.end
extrude "Extrusion15" cut sketch "Skizze20" against normal blind 0.5 contours L2 L15 L8 L13 | L13 L6 L15 L3 | L13 L6 L7 L8 | L8 L15 L6 L13 | L8 L9 L6 L15
ref_plane "Arbeitsebene3" through (0, 0, 20.1) normal (0, 0, -1) x (-1, 0, 0)
sketch "Skizze21" plane through (-20, -20, 0) normal (0, -1, 0) x (1, 0, 0)
  line L0 (30, 19.75) -> (30, 20.25) projected
  line L1 (30, 20.25) -> (20.25, 20.25) projected
  line L2 (20.25, 20.25) -> (20.25, 30.1) projected
  line L3 (20.25, 30.1) -> (19.75, 30.1) projected
  line L4 (19.75, 30.1) -> (19.75, 20.25) projected
  line L5 (19.75, 20.25) -> (10, 20.25) projected
  line L6 (10, 20.25) -> (10, 19.75) projected
  line L7 (10, 19.75) -> (19.75, 19.75) projected
  line L8 (19.75, 19.75) -> (19.75, 9.9) projected
  line L9 (19.75, 9.9) -> (20.25, 9.9) projected
  line L10 (20.25, 9.9) -> (20.25, 19.75) projected
  line L11 (20.25, 19.75) -> (30, 19.75) projected
  line L12 (0, 40) -> (0, 0) projected
  line L13 (0, 40) -> (70, 40) projected
  line L14 (70, 0) -> (70, 40) projected
  line L15 (0, 0) -> (70, 0) projected
  point P0 (20, 0)
extrude "Extrusion16" cut sketch "Skizze21" against normal blind 0.5 contours L11 L10 L9 L8 L7 L6 L5 L4 L3 L2 L1 L0
ref_plane "Arbeitsebene4" through (0.1, -20, 70) normal (-1, 0, 0) x (0, 0, 1)
